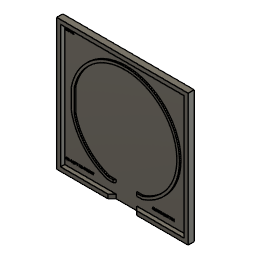
pin_grid_center_wafer_jig (Autodesk Fusion 360 design; units mm, degrees)
part number: 2026-08-08-01-37-12-857
Autodesk Fusion 360 part; units mm, degrees
ref_plane "WorkPlane1" through (0, 0, 2) normal (0, 0, 1) x (1, 0, 0)
ref_plane "WorkPlane2" through (0, 0, 3.7) normal (0, 0, 1) x (1, 0, 0)
ref_plane "WorkPlane3" through (0, 0, 6.2) normal (0, 0, 1) x (1, 0, 0)
ref_plane "WorkPlane4" through (0, 0, -5) normal (0, 0, 1) x (1, 0, 0)
ref_plane "WorkPlane5" through (0, 0, -4) normal (0, 0, 1) x (1, 0, 0)
sketch "128 mm Square Wafer Platform Sketch" plane through (0, 0, 0) normal (0, 0, 1) x (1, 0, 0)
  line L0 (-56.71, -68.95) -> (71.29, -68.95)
  line L1 (71.29, -68.95) -> (71.29, 59.05)
  line L2 (71.29, 59.05) -> (-56.71, 59.05)
  line L3 (-56.71, 59.05) -> (-56.71, -68.95)
extrude "128 mm Square Wafer Platform" add sketch "128 mm Square Wafer Platform Sketch" along normal blind 2
sketch "4 x 4 mm Perimeter Reinforcement Bar Sketch" plane through (0, 0, 2) normal (0, 0, 1) x (1, 0, 0)
  line L0 (-56.71, -68.95) -> (71.29, -68.95)
  line L1 (71.29, -68.95) -> (71.29, 59.05)
  line L2 (71.29, 59.05) -> (-56.71, 59.05)
  line L3 (-56.71, 59.05) -> (-56.71, -68.95)
  line L4 (-52.71, -64.95) -> (67.29, -64.95)
  line L5 (67.29, -64.95) -> (67.29, 55.05)
  line L6 (67.29, 55.05) -> (-52.71, 55.05)
  line L7 (-52.71, 55.05) -> (-52.71, -64.95)
extrude "4 x 4 mm Perimeter Reinforcement Bar" add sketch "4 x 4 mm Perimeter Reinforcement Bar Sketch" along normal blind 4
sketch "20 mm Outer Bar Tweezer Notch with 45 Degree Sides Lower Sketch" plane through (0, 0, 2) normal (0, 0, 1) x (1, 0, 0)
  line L0 (-2.71, -69.05) -> (17.29, -69.05)
  line L1 (17.29, -69.05) -> (17.29, -64.85)
  line L2 (17.29, -64.85) -> (-2.71, -64.85)
  line L3 (-2.71, -64.85) -> (-2.71, -69.05)
sketch "20 mm Outer Bar Tweezer Notch with 45 Degree Sides Upper Sketch" plane through (0, 0, 6.2) normal (0, 0, 1) x (1, 0, 0)
  line L0 (-6.91, -73.25) -> (21.49, -73.25)
  line L1 (21.49, -73.25) -> (21.49, -60.65)
  line L2 (21.49, -60.65) -> (-6.91, -60.65)
  line L3 (-6.91, -60.65) -> (-6.91, -73.25)
loft "20 mm Outer Bar Tweezer Notch with 45 Degree Sides" cut profiles "20 mm Outer Bar Tweezer Notch with 45 Degree Sides Lower Sketch", "20 mm Outer Bar Tweezer Notch with 45 Degree Sides Upper Sketch" section 1 section 2
sketch "1.5 mm Raised Wafer Nest Sketch" plane through (0, 0, 2) normal (0, 0, 1) x (1, 0, 0)
  line L0 (60.29, -4.95) -> (60.2577, -3.1003)
  line L1 (60.2577, -3.1003) -> (60.1609, -1.2529)
  line L2 (60.1609, -1.2529) -> (59.9997, 0.59)
  line L3 (59.9997, 0.59) -> (59.7742, 2.4262)
  line L4 (59.7742, 2.4262) -> (59.4848, 4.2534)
  line L5 (59.4848, 4.2534) -> (59.1318, 6.0693)
  line L6 (59.1318, 6.0693) -> (58.7157, 7.8719)
  line L7 (58.7157, 7.8719) -> (58.2369, 9.6588)
  line L8 (58.2369, 9.6588) -> (57.696, 11.4279)
  line L9 (57.696, 11.4279) -> (57.0937, 13.1771)
  line L10 (57.0937, 13.1771) -> (56.4307, 14.9041)
  line L11 (56.4307, 14.9041) -> (55.7079, 16.607)
  line L12 (55.7079, 16.607) -> (54.9261, 18.2837)
  line L13 (54.9261, 18.2837) -> (54.0862, 19.932)
  line L14 (54.0862, 19.932) -> (53.1893, 21.55)
  line L15 (53.1893, 21.55) -> (52.2365, 23.1357)
  line L16 (52.2365, 23.1357) -> (51.229, 24.6872)
  line L17 (51.229, 24.6872) -> (50.1679, 26.2026)
  line L18 (50.1679, 26.2026) -> (49.0546, 27.6801)
  line L19 (49.0546, 27.6801) -> (47.8904, 29.1177)
  line L20 (47.8904, 29.1177) -> (46.6767, 30.5139)
  line L21 (46.6767, 30.5139) -> (45.415, 31.8669)
  line L22 (45.415, 31.8669) -> (44.1069, 33.175)
  line L23 (44.1069, 33.175) -> (42.7539, 34.4367)
  line L24 (42.7539, 34.4367) -> (41.3577, 35.6504)
  line L25 (41.3577, 35.6504) -> (39.9201, 36.8146)
  line L26 (39.9201, 36.8146) -> (38.4426, 37.9279)
  line L27 (38.4426, 37.9279) -> (36.9272, 38.989)
  line L28 (36.9272, 38.989) -> (35.3757, 39.9965)
  line L29 (35.3757, 39.9965) -> (33.79, 40.9493)
  line L30 (33.79, 40.9493) -> (32.172, 41.8462)
  line L31 (32.172, 41.8462) -> (30.5237, 42.6861)
  line L32 (30.5237, 42.6861) -> (28.847, 43.4679)
  line L33 (28.847, 43.4679) -> (27.1441, 44.1907)
  line L34 (27.1441, 44.1907) -> (25.4171, 44.8537)
  line L35 (25.4171, 44.8537) -> (23.6679, 45.456)
  line L36 (23.6679, 45.456) -> (21.8988, 45.9969)
  line L37 (21.8988, 45.9969) -> (20.1119, 46.4757)
  line L38 (20.1119, 46.4757) -> (18.3093, 46.8918)
  line L39 (18.3093, 46.8918) -> (16.4934, 47.2448)
  line L40 (16.4934, 47.2448) -> (14.6662, 47.5342)
  line L41 (14.6662, 47.5342) -> (12.83, 47.7597)
  line L42 (12.83, 47.7597) -> (10.9871, 47.9209)
  line L43 (10.9871, 47.9209) -> (9.1397, 48.0177)
  line L44 (9.1397, 48.0177) -> (7.29, 48.05)
  line L45 (7.29, 48.05) -> (5.4403, 48.0177)
  line L46 (5.4403, 48.0177) -> (3.5929, 47.9209)
  line L47 (3.5929, 47.9209) -> (1.75, 47.7597)
  line L48 (1.75, 47.7597) -> (-0.0862, 47.5342)
  line L49 (-0.0862, 47.5342) -> (-1.9134, 47.2448)
  line L50 (-1.9134, 47.2448) -> (-3.7293, 46.8918)
  line L51 (-3.7293, 46.8918) -> (-5.5319, 46.4757)
  line L52 (-5.5319, 46.4757) -> (-7.3188, 45.9969)
  line L53 (-7.3188, 45.9969) -> (-9.0879, 45.456)
  line L54 (-9.0879, 45.456) -> (-10.8371, 44.8537)
  line L55 (-10.8371, 44.8537) -> (-12.5641, 44.1907)
  line L56 (-12.5641, 44.1907) -> (-14.267, 43.4679)
  line L57 (-14.267, 43.4679) -> (-15.9437, 42.6861)
  line L58 (-15.9437, 42.6861) -> (-17.592, 41.8462)
  line L59 (-17.592, 41.8462) -> (-19.21, 40.9493)
  line L60 (-19.21, 40.9493) -> (-20.7957, 39.9965)
  line L61 (-20.7957, 39.9965) -> (-22.3472, 38.989)
  line L62 (-22.3472, 38.989) -> (-23.8626, 37.9279)
  line L63 (-23.8626, 37.9279) -> (-25.3401, 36.8146)
  line L64 (-25.3401, 36.8146) -> (-26.7777, 35.6504)
  line L65 (-26.7777, 35.6504) -> (-28.1739, 34.4367)
  line L66 (-28.1739, 34.4367) -> (-29.5269, 33.175)
  line L67 (-29.5269, 33.175) -> (-30.835, 31.8669)
  line L68 (-30.835, 31.8669) -> (-32.0967, 30.5139)
  line L69 (-32.0967, 30.5139) -> (-33.3104, 29.1177)
  line L70 (-33.3104, 29.1177) -> (-34.4746, 27.6801)
  line L71 (-34.4746, 27.6801) -> (-35.5879, 26.2026)
  line L72 (-35.5879, 26.2026) -> (-36.649, 24.6872)
  line L73 (-36.649, 24.6872) -> (-37.6565, 23.1357)
  line L74 (-37.6565, 23.1357) -> (-38.6093, 21.55)
  line L75 (-38.6093, 21.55) -> (-39.5062, 19.932)
  line L76 (-39.5062, 19.932) -> (-40.3461, 18.2837)
  line L77 (-40.3461, 18.2837) -> (-41.1279, 16.607)
  line L78 (-41.1279, 16.607) -> (-41.8507, 14.9041)
  line L79 (-41.8507, 14.9041) -> (-42.5137, 13.1771)
  line L80 (-42.5137, 13.1771) -> (-43.116, 11.4279)
  line L81 (-43.116, 11.4279) -> (-43.6569, 9.6588)
  line L82 (-43.6569, 9.6588) -> (-44.1357, 7.8719)
  line L83 (-44.1357, 7.8719) -> (-44.5518, 6.0693)
  line L84 (-44.5518, 6.0693) -> (-44.8933, 4.3124)
  line L85 (-44.8933, 4.3124) -> (-44.8933, -14.2124)
  line L86 (-44.8933, -14.2124) -> (-44.5518, -15.9693)
  line L87 (-44.5518, -15.9693) -> (-44.1357, -17.7719)
  line L88 (-44.1357, -17.7719) -> (-43.6569, -19.5588)
  line L89 (-43.6569, -19.5588) -> (-43.116, -21.3279)
  line L90 (-43.116, -21.3279) -> (-42.5137, -23.0771)
  line L91 (-42.5137, -23.0771) -> (-41.8507, -24.8041)
  line L92 (-41.8507, -24.8041) -> (-41.1279, -26.507)
  line L93 (-41.1279, -26.507) -> (-40.3461, -28.1837)
  line L94 (-40.3461, -28.1837) -> (-39.5062, -29.832)
  line L95 (-39.5062, -29.832) -> (-38.6093, -31.45)
  line L96 (-38.6093, -31.45) -> (-37.6565, -33.0357)
  line L97 (-37.6565, -33.0357) -> (-36.649, -34.5872)
  line L98 (-36.649, -34.5872) -> (-35.5879, -36.1026)
  line L99 (-35.5879, -36.1026) -> (-34.4746, -37.5801)
  line L100 (-34.4746, -37.5801) -> (-33.3104, -39.0177)
  line L101 (-33.3104, -39.0177) -> (-32.0967, -40.4139)
  line L102 (-32.0967, -40.4139) -> (-30.835, -41.7669)
  line L103 (-30.835, -41.7669) -> (-29.5269, -43.075)
  line L104 (-29.5269, -43.075) -> (-28.1739, -44.3367)
  line L105 (-28.1739, -44.3367) -> (-26.7777, -45.5504)
  line L106 (-26.7777, -45.5504) -> (-25.3401, -46.7146)
  line L107 (-25.3401, -46.7146) -> (-23.8626, -47.8279)
  line L108 (-23.8626, -47.8279) -> (-22.3472, -48.889)
  line L109 (-22.3472, -48.889) -> (-20.7957, -49.8965)
  line L110 (-20.7957, -49.8965) -> (-19.21, -50.8493)
  line L111 (-19.21, -50.8493) -> (-17.592, -51.7462)
  line L112 (-17.592, -51.7462) -> (-15.9437, -52.5861)
  line L113 (-15.9437, -52.5861) -> (-14.267, -53.3679)
  line L114 (-14.267, -53.3679) -> (-12.5641, -54.0907)
  line L115 (-12.5641, -54.0907) -> (-10.8371, -54.7537)
  line L116 (-10.8371, -54.7537) -> (-9.4373, -55.2357)
  line L117 (-9.4373, -55.2357) -> (24.0173, -55.2357)
  line L118 (24.0173, -55.2357) -> (25.4171, -54.7537)
  line L119 (25.4171, -54.7537) -> (27.1441, -54.0907)
  line L120 (27.1441, -54.0907) -> (28.847, -53.3679)
  line L121 (28.847, -53.3679) -> (30.5237, -52.5861)
  line L122 (30.5237, -52.5861) -> (32.172, -51.7462)
  line L123 (32.172, -51.7462) -> (33.79, -50.8493)
  line L124 (33.79, -50.8493) -> (35.3757, -49.8965)
  line L125 (35.3757, -49.8965) -> (36.9272, -48.889)
  line L126 (36.9272, -48.889) -> (38.4426, -47.8279)
  line L127 (38.4426, -47.8279) -> (39.9201, -46.7146)
  line L128 (39.9201, -46.7146) -> (41.3577, -45.5504)
  line L129 (41.3577, -45.5504) -> (42.7539, -44.3367)
  line L130 (42.7539, -44.3367) -> (44.1069, -43.075)
  line L131 (44.1069, -43.075) -> (45.415, -41.7669)
  line L132 (45.415, -41.7669) -> (46.6767, -40.4139)
  line L133 (46.6767, -40.4139) -> (47.8904, -39.0177)
  line L134 (47.8904, -39.0177) -> (49.0546, -37.5801)
  line L135 (49.0546, -37.5801) -> (50.1679, -36.1026)
  line L136 (50.1679, -36.1026) -> (51.229, -34.5872)
  line L137 (51.229, -34.5872) -> (52.2365, -33.0357)
  line L138 (52.2365, -33.0357) -> (53.1893, -31.45)
  line L139 (53.1893, -31.45) -> (54.0862, -29.832)
  line L140 (54.0862, -29.832) -> (54.9261, -28.1837)
  line L141 (54.9261, -28.1837) -> (55.7079, -26.507)
  line L142 (55.7079, -26.507) -> (56.4307, -24.8041)
  line L143 (56.4307, -24.8041) -> (57.0937, -23.0771)
  line L144 (57.0937, -23.0771) -> (57.696, -21.3279)
  line L145 (57.696, -21.3279) -> (58.2369, -19.5588)
  line L146 (58.2369, -19.5588) -> (58.7157, -17.7719)
  line L147 (58.7157, -17.7719) -> (59.1318, -15.9693)
  line L148 (59.1318, -15.9693) -> (59.4848, -14.1534)
  line L149 (59.4848, -14.1534) -> (59.7742, -12.3262)
  line L150 (59.7742, -12.3262) -> (59.9997, -10.49)
  line L151 (59.9997, -10.49) -> (60.1609, -8.6471)
  line L152 (60.1609, -8.6471) -> (60.2577, -6.7997)
  line L153 (60.2577, -6.7997) -> (60.29, -4.95)
extrude "1.5 mm Raised Wafer Nest" add sketch "1.5 mm Raised Wafer Nest Sketch" along normal blind 1.5
sketch "Final Wafer Pocket Clearance Sketch" plane through (0, 0, 2) normal (0, 0, 1) x (1, 0, 0)
  line L0 (57.79, -4.95) -> (57.7592, -3.1876)
  line L1 (57.7592, -3.1876) -> (57.667, -1.4273)
  line L2 (57.667, -1.4273) -> (57.5134, 0.3287)
  line L3 (57.5134, 0.3287) -> (57.2985, 2.0782)
  line L4 (57.2985, 2.0782) -> (57.0228, 3.8192)
  line L5 (57.0228, 3.8192) -> (56.6865, 5.5495)
  line L6 (56.6865, 5.5495) -> (56.2899, 7.2671)
  line L7 (56.2899, 7.2671) -> (55.8337, 8.9697)
  line L8 (55.8337, 8.9697) -> (55.3184, 10.6554)
  line L9 (55.3184, 10.6554) -> (54.7445, 12.322)
  line L10 (54.7445, 12.322) -> (54.1128, 13.9676)
  line L11 (54.1128, 13.9676) -> (53.424, 15.5902)
  line L12 (53.424, 15.5902) -> (52.6791, 17.1877)
  line L13 (52.6791, 17.1877) -> (51.8789, 18.7583)
  line L14 (51.8789, 18.7583) -> (51.0243, 20.3)
  line L15 (51.0243, 20.3) -> (50.1164, 21.8109)
  line L16 (50.1164, 21.8109) -> (49.1564, 23.2892)
  line L17 (49.1564, 23.2892) -> (48.1454, 24.7332)
  line L18 (48.1454, 24.7332) -> (47.0845, 26.1409)
  line L19 (47.0845, 26.1409) -> (45.9752, 27.5108)
  line L20 (45.9752, 27.5108) -> (44.8188, 28.8411)
  line L21 (44.8188, 28.8411) -> (43.6167, 30.1302)
  line L22 (43.6167, 30.1302) -> (42.3702, 31.3767)
  line L23 (42.3702, 31.3767) -> (41.0811, 32.5788)
  line L24 (41.0811, 32.5788) -> (39.7508, 33.7352)
  line L25 (39.7508, 33.7352) -> (38.3809, 34.8445)
  line L26 (38.3809, 34.8445) -> (36.9732, 35.9054)
  line L27 (36.9732, 35.9054) -> (35.5292, 36.9164)
  line L28 (35.5292, 36.9164) -> (34.0509, 37.8764)
  line L29 (34.0509, 37.8764) -> (32.54, 38.7843)
  line L30 (32.54, 38.7843) -> (30.9983, 39.6389)
  line L31 (30.9983, 39.6389) -> (29.4277, 40.4391)
  line L32 (29.4277, 40.4391) -> (27.8302, 41.184)
  line L33 (27.8302, 41.184) -> (26.2076, 41.8728)
  line L34 (26.2076, 41.8728) -> (24.562, 42.5045)
  line L35 (24.562, 42.5045) -> (22.8954, 43.0784)
  line L36 (22.8954, 43.0784) -> (21.2097, 43.5937)
  line L37 (21.2097, 43.5937) -> (19.5071, 44.0499)
  line L38 (19.5071, 44.0499) -> (17.7895, 44.4465)
  line L39 (17.7895, 44.4465) -> (16.0592, 44.7828)
  line L40 (16.0592, 44.7828) -> (14.3182, 45.0585)
  line L41 (14.3182, 45.0585) -> (12.5687, 45.2734)
  line L42 (12.5687, 45.2734) -> (10.8127, 45.427)
  line L43 (10.8127, 45.427) -> (9.0524, 45.5192)
  line L44 (9.0524, 45.5192) -> (7.29, 45.55)
  line L45 (7.29, 45.55) -> (5.5276, 45.5192)
  line L46 (5.5276, 45.5192) -> (3.7673, 45.427)
  line L47 (3.7673, 45.427) -> (2.0113, 45.2734)
  line L48 (2.0113, 45.2734) -> (0.2618, 45.0585)
  line L49 (0.2618, 45.0585) -> (-1.4792, 44.7828)
  line L50 (-1.4792, 44.7828) -> (-3.2095, 44.4465)
  line L51 (-3.2095, 44.4465) -> (-4.9271, 44.0499)
  line L52 (-4.9271, 44.0499) -> (-6.6297, 43.5937)
  line L53 (-6.6297, 43.5937) -> (-8.3154, 43.0784)
  line L54 (-8.3154, 43.0784) -> (-9.982, 42.5045)
  line L55 (-9.982, 42.5045) -> (-11.6276, 41.8728)
  line L56 (-11.6276, 41.8728) -> (-13.2502, 41.184)
  line L57 (-13.2502, 41.184) -> (-14.8477, 40.4391)
  line L58 (-14.8477, 40.4391) -> (-16.4183, 39.6389)
  line L59 (-16.4183, 39.6389) -> (-17.96, 38.7843)
  line L60 (-17.96, 38.7843) -> (-19.4709, 37.8764)
  line L61 (-19.4709, 37.8764) -> (-20.9492, 36.9164)
  line L62 (-20.9492, 36.9164) -> (-22.3932, 35.9054)
  line L63 (-22.3932, 35.9054) -> (-23.8009, 34.8445)
  line L64 (-23.8009, 34.8445) -> (-25.1708, 33.7352)
  line L65 (-25.1708, 33.7352) -> (-26.5011, 32.5788)
  line L66 (-26.5011, 32.5788) -> (-27.7902, 31.3767)
  line L67 (-27.7902, 31.3767) -> (-29.0367, 30.1302)
  line L68 (-29.0367, 30.1302) -> (-30.2388, 28.8411)
  line L69 (-30.2388, 28.8411) -> (-31.3952, 27.5108)
  line L70 (-31.3952, 27.5108) -> (-32.5045, 26.1409)
  line L71 (-32.5045, 26.1409) -> (-33.5654, 24.7332)
  line L72 (-33.5654, 24.7332) -> (-34.5764, 23.2892)
  line L73 (-34.5764, 23.2892) -> (-35.5364, 21.8109)
  line L74 (-35.5364, 21.8109) -> (-36.4443, 20.3)
  line L75 (-36.4443, 20.3) -> (-37.2989, 18.7583)
  line L76 (-37.2989, 18.7583) -> (-38.0991, 17.1877)
  line L77 (-38.0991, 17.1877) -> (-38.844, 15.5902)
  line L78 (-38.844, 15.5902) -> (-39.5328, 13.9676)
  line L79 (-39.5328, 13.9676) -> (-40.1645, 12.322)
  line L80 (-40.1645, 12.322) -> (-40.7384, 10.6554)
  line L81 (-40.7384, 10.6554) -> (-41.2537, 8.9697)
  line L82 (-41.2537, 8.9697) -> (-41.7099, 7.2671)
  line L83 (-41.7099, 7.2671) -> (-41.9933, 6.0395)
  line L84 (-41.9933, 6.0395) -> (-41.9933, -15.9395)
  line L85 (-41.9933, -15.9395) -> (-41.7099, -17.1671)
  line L86 (-41.7099, -17.1671) -> (-41.2537, -18.8697)
  line L87 (-41.2537, -18.8697) -> (-40.7384, -20.5554)
  line L88 (-40.7384, -20.5554) -> (-40.1645, -22.222)
  line L89 (-40.1645, -22.222) -> (-39.5328, -23.8676)
  line L90 (-39.5328, -23.8676) -> (-38.844, -25.4902)
  line L91 (-38.844, -25.4902) -> (-38.0991, -27.0877)
  line L92 (-38.0991, -27.0877) -> (-37.2989, -28.6583)
  line L93 (-37.2989, -28.6583) -> (-36.4443, -30.2)
  line L94 (-36.4443, -30.2) -> (-35.5364, -31.7109)
  line L95 (-35.5364, -31.7109) -> (-34.5764, -33.1892)
  line L96 (-34.5764, -33.1892) -> (-33.5654, -34.6332)
  line L97 (-33.5654, -34.6332) -> (-32.5045, -36.0409)
  line L98 (-32.5045, -36.0409) -> (-31.3952, -37.4108)
  line L99 (-31.3952, -37.4108) -> (-30.2388, -38.7411)
  line L100 (-30.2388, -38.7411) -> (-29.0367, -40.0302)
  line L101 (-29.0367, -40.0302) -> (-27.7902, -41.2767)
  line L102 (-27.7902, -41.2767) -> (-26.5011, -42.4788)
  line L103 (-26.5011, -42.4788) -> (-25.1708, -43.6352)
  line L104 (-25.1708, -43.6352) -> (-23.8009, -44.7445)
  line L105 (-23.8009, -44.7445) -> (-22.3932, -45.8054)
  line L106 (-22.3932, -45.8054) -> (-20.9492, -46.8164)
  line L107 (-20.9492, -46.8164) -> (-19.4709, -47.7764)
  line L108 (-19.4709, -47.7764) -> (-17.96, -48.6843)
  line L109 (-17.96, -48.6843) -> (-16.4183, -49.5389)
  line L110 (-16.4183, -49.5389) -> (-14.8477, -50.3391)
  line L111 (-14.8477, -50.3391) -> (-13.2502, -51.084)
  line L112 (-13.2502, -51.084) -> (-11.6276, -51.7728)
  line L113 (-11.6276, -51.7728) -> (-9.982, -52.4045)
  line L114 (-9.982, -52.4045) -> (-9.0201, -52.7357)
  line L115 (-9.0201, -52.7357) -> (23.6001, -52.7357)
  line L116 (23.6001, -52.7357) -> (24.562, -52.4045)
  line L117 (24.562, -52.4045) -> (26.2076, -51.7728)
  line L118 (26.2076, -51.7728) -> (27.8302, -51.084)
  line L119 (27.8302, -51.084) -> (29.4277, -50.3391)
  line L120 (29.4277, -50.3391) -> (30.9983, -49.5389)
  line L121 (30.9983, -49.5389) -> (32.54, -48.6843)
  line L122 (32.54, -48.6843) -> (34.0509, -47.7764)
  line L123 (34.0509, -47.7764) -> (35.5292, -46.8164)
  line L124 (35.5292, -46.8164) -> (36.9732, -45.8054)
  line L125 (36.9732, -45.8054) -> (38.3809, -44.7445)
  line L126 (38.3809, -44.7445) -> (39.7508, -43.6352)
  line L127 (39.7508, -43.6352) -> (41.0811, -42.4788)
  line L128 (41.0811, -42.4788) -> (42.3702, -41.2767)
  line L129 (42.3702, -41.2767) -> (43.6167, -40.0302)
  line L130 (43.6167, -40.0302) -> (44.8188, -38.7411)
  line L131 (44.8188, -38.7411) -> (45.9752, -37.4108)
  line L132 (45.9752, -37.4108) -> (47.0845, -36.0409)
  line L133 (47.0845, -36.0409) -> (48.1454, -34.6332)
  line L134 (48.1454, -34.6332) -> (49.1564, -33.1892)
  line L135 (49.1564, -33.1892) -> (50.1164, -31.7109)
  line L136 (50.1164, -31.7109) -> (51.0243, -30.2)
  line L137 (51.0243, -30.2) -> (51.8789, -28.6583)
  line L138 (51.8789, -28.6583) -> (52.6791, -27.0877)
  line L139 (52.6791, -27.0877) -> (53.424, -25.4902)
  line L140 (53.424, -25.4902) -> (54.1128, -23.8676)
  line L141 (54.1128, -23.8676) -> (54.7445, -22.222)
  line L142 (54.7445, -22.222) -> (55.3184, -20.5554)
  line L143 (55.3184, -20.5554) -> (55.8337, -18.8697)
  line L144 (55.8337, -18.8697) -> (56.2899, -17.1671)
  line L145 (56.2899, -17.1671) -> (56.6865, -15.4495)
  line L146 (56.6865, -15.4495) -> (57.0228, -13.7192)
  line L147 (57.0228, -13.7192) -> (57.2985, -11.9782)
  line L148 (57.2985, -11.9782) -> (57.5134, -10.2287)
  line L149 (57.5134, -10.2287) -> (57.667, -8.4727)
  line L150 (57.667, -8.4727) -> (57.7592, -6.7124)
  line L151 (57.7592, -6.7124) -> (57.79, -4.95)
extrude "Final Wafer Pocket Clearance" cut sketch "Final Wafer Pocket Clearance Sketch" along normal blind 1.6
sketch "20 mm Pickup Opening with 45 Degree Bevel Lower Sketch" plane through (0, 0, 2) normal (0, 0, 1) x (1, 0, 0)
  line L0 (-2.71, -55.2357) -> (-2.71, -52.2357)
  line L1 (-2.71, -52.2357) -> (-2.6471, -51.1161)
  line L2 (-2.6471, -51.1161) -> (-2.4593, -50.0105)
  line L3 (-2.4593, -50.0105) -> (-2.1488, -48.9329)
  line L4 (-2.1488, -48.9329) -> (-1.7197, -47.8969)
  line L5 (-1.7197, -47.8969) -> (-1.1772, -46.9154)
  line L6 (-1.1772, -46.9154) -> (-0.5283, -46.0008)
  line L7 (-0.5283, -46.0008) -> (0.2189, -45.1646)
  line L8 (0.2189, -45.1646) -> (1.0551, -44.4174)
  line L9 (1.0551, -44.4174) -> (1.9697, -43.7685)
  line L10 (1.9697, -43.7685) -> (2.9512, -43.226)
  line L11 (2.9512, -43.226) -> (3.9872, -42.7969)
  line L12 (3.9872, -42.7969) -> (5.0648, -42.4864)
  line L13 (5.0648, -42.4864) -> (6.1704, -42.2986)
  line L14 (6.1704, -42.2986) -> (7.29, -42.2357)
  line L15 (7.29, -42.2357) -> (8.4096, -42.2986)
  line L16 (8.4096, -42.2986) -> (9.5152, -42.4864)
  line L17 (9.5152, -42.4864) -> (10.5928, -42.7969)
  line L18 (10.5928, -42.7969) -> (11.6288, -43.226)
  line L19 (11.6288, -43.226) -> (12.6103, -43.7685)
  line L20 (12.6103, -43.7685) -> (13.5249, -44.4174)
  line L21 (13.5249, -44.4174) -> (14.3611, -45.1646)
  line L22 (14.3611, -45.1646) -> (15.1083, -46.0008)
  line L23 (15.1083, -46.0008) -> (15.7572, -46.9154)
  line L24 (15.7572, -46.9154) -> (16.2997, -47.8969)
  line L25 (16.2997, -47.8969) -> (16.7288, -48.9329)
  line L26 (16.7288, -48.9329) -> (17.0393, -50.0105)
  line L27 (17.0393, -50.0105) -> (17.2271, -51.1161)
  line L28 (17.2271, -51.1161) -> (17.29, -52.2357)
  line L29 (17.29, -52.2357) -> (17.29, -55.2357)
  line L30 (17.29, -55.2357) -> (17.2271, -56.3553)
  line L31 (17.2271, -56.3553) -> (17.0393, -57.4609)
  line L32 (17.0393, -57.4609) -> (16.7288, -58.5385)
  line L33 (16.7288, -58.5385) -> (16.2997, -59.5745)
  line L34 (16.2997, -59.5745) -> (15.7572, -60.556)
  line L35 (15.7572, -60.556) -> (15.1083, -61.4706)
  line L36 (15.1083, -61.4706) -> (14.3611, -62.3068)
  line L37 (14.3611, -62.3068) -> (13.5249, -63.054)
  line L38 (13.5249, -63.054) -> (12.6103, -63.7029)
  line L39 (12.6103, -63.7029) -> (11.6288, -64.2454)
  line L40 (11.6288, -64.2454) -> (10.5928, -64.6745)
  line L41 (10.5928, -64.6745) -> (9.5152, -64.985)
  line L42 (9.5152, -64.985) -> (8.4096, -65.1728)
  line L43 (8.4096, -65.1728) -> (7.29, -65.2357)
  line L44 (7.29, -65.2357) -> (6.1704, -65.1728)
  line L45 (6.1704, -65.1728) -> (5.0648, -64.985)
  line L46 (5.0648, -64.985) -> (3.9872, -64.6745)
  line L47 (3.9872, -64.6745) -> (2.9512, -64.2454)
  line L48 (2.9512, -64.2454) -> (1.9697, -63.7029)
  line L49 (1.9697, -63.7029) -> (1.0551, -63.054)
  line L50 (1.0551, -63.054) -> (0.2189, -62.3068)
  line L51 (0.2189, -62.3068) -> (-0.5283, -61.4706)
  line L52 (-0.5283, -61.4706) -> (-1.1772, -60.556)
  line L53 (-1.1772, -60.556) -> (-1.7197, -59.5745)
  line L54 (-1.7197, -59.5745) -> (-2.1488, -58.5385)
  line L55 (-2.1488, -58.5385) -> (-2.4593, -57.4609)
  line L56 (-2.4593, -57.4609) -> (-2.6471, -56.3553)
  line L57 (-2.6471, -56.3553) -> (-2.71, -55.2357)
sketch "20 mm Pickup Opening with 45 Degree Bevel Upper Sketch" plane through (0, 0, 3.7) normal (0, 0, 1) x (1, 0, 0)
  line L0 (-4.41, -56.9357) -> (-4.41, -50.5357)
  line L1 (-4.41, -50.5357) -> (-4.3364, -49.2257)
  line L2 (-4.3364, -49.2257) -> (-4.1167, -47.9322)
  line L3 (-4.1167, -47.9322) -> (-3.7534, -46.6714)
  line L4 (-3.7534, -46.6714) -> (-3.2513, -45.4593)
  line L5 (-3.2513, -45.4593) -> (-2.6167, -44.3109)
  line L6 (-2.6167, -44.3109) -> (-1.8574, -43.2409)
  line L7 (-1.8574, -43.2409) -> (-0.9831, -42.2626)
  line L8 (-0.9831, -42.2626) -> (-0.0048, -41.3883)
  line L9 (-0.0048, -41.3883) -> (1.0652, -40.629)
  line L10 (1.0652, -40.629) -> (2.2136, -39.9944)
  line L11 (2.2136, -39.9944) -> (3.4257, -39.4923)
  line L12 (3.4257, -39.4923) -> (4.6865, -39.129)
  line L13 (4.6865, -39.129) -> (5.98, -38.9093)
  line L14 (5.98, -38.9093) -> (7.29, -38.8357)
  line L15 (7.29, -38.8357) -> (8.6, -38.9093)
  line L16 (8.6, -38.9093) -> (9.8935, -39.129)
  line L17 (9.8935, -39.129) -> (11.1543, -39.4923)
  line L18 (11.1543, -39.4923) -> (12.3664, -39.9944)
  line L19 (12.3664, -39.9944) -> (13.5148, -40.629)
  line L20 (13.5148, -40.629) -> (14.5848, -41.3883)
  line L21 (14.5848, -41.3883) -> (15.5631, -42.2626)
  line L22 (15.5631, -42.2626) -> (16.4374, -43.2409)
  line L23 (16.4374, -43.2409) -> (17.1967, -44.3109)
  line L24 (17.1967, -44.3109) -> (17.8313, -45.4593)
  line L25 (17.8313, -45.4593) -> (18.3334, -46.6714)
  line L26 (18.3334, -46.6714) -> (18.6967, -47.9322)
  line L27 (18.6967, -47.9322) -> (18.9164, -49.2257)
  line L28 (18.9164, -49.2257) -> (18.99, -50.5357)
  line L29 (18.99, -50.5357) -> (18.99, -56.9357)
  line L30 (18.99, -56.9357) -> (18.9164, -58.2457)
  line L31 (18.9164, -58.2457) -> (18.6967, -59.5392)
  line L32 (18.6967, -59.5392) -> (18.3334, -60.8)
  line L33 (18.3334, -60.8) -> (17.8313, -62.0121)
  line L34 (17.8313, -62.0121) -> (17.1967, -63.1605)
  line L35 (17.1967, -63.1605) -> (16.4374, -64.2305)
  line L36 (16.4374, -64.2305) -> (15.5631, -65.2089)
  line L37 (15.5631, -65.2089) -> (14.5848, -66.0831)
  line L38 (14.5848, -66.0831) -> (13.5148, -66.8424)
  line L39 (13.5148, -66.8424) -> (12.3664, -67.477)
  line L40 (12.3664, -67.477) -> (11.1543, -67.9791)
  line L41 (11.1543, -67.9791) -> (9.8935, -68.3424)
  line L42 (9.8935, -68.3424) -> (8.6, -68.5621)
  line L43 (8.6, -68.5621) -> (7.29, -68.6357)
  line L44 (7.29, -68.6357) -> (5.98, -68.5621)
  line L45 (5.98, -68.5621) -> (4.6865, -68.3424)
  line L46 (4.6865, -68.3424) -> (3.4257, -67.9791)
  line L47 (3.4257, -67.9791) -> (2.2136, -67.477)
  line L48 (2.2136, -67.477) -> (1.0652, -66.8424)
  line L49 (1.0652, -66.8424) -> (-0.0048, -66.0831)
  line L50 (-0.0048, -66.0831) -> (-0.9831, -65.2089)
  line L51 (-0.9831, -65.2089) -> (-1.8574, -64.2305)
  line L52 (-1.8574, -64.2305) -> (-2.6167, -63.1605)
  line L53 (-2.6167, -63.1605) -> (-3.2513, -62.0121)
  line L54 (-3.2513, -62.0121) -> (-3.7534, -60.8)
  line L55 (-3.7534, -60.8) -> (-4.1167, -59.5392)
  line L56 (-4.1167, -59.5392) -> (-4.3364, -58.2457)
  line L57 (-4.3364, -58.2457) -> (-4.41, -56.9357)
loft "20 mm Pickup Opening with 45 Degree Bevel" cut profiles "20 mm Pickup Opening with 45 Degree Bevel Lower Sketch", "20 mm Pickup Opening with 45 Degree Bevel Upper Sketch" section 1 section 2
sketch "Outer Front Left Pin Cylinder Sketch" plane through (0, 0, -4) normal (0, 0, 1) x (1, 0, 0)
  circle A0 centre (-50.8, -50.8) radius 2.35
extrude "Outer Front Left 4.7 mm Pin" add sketch "Outer Front Left Pin Cylinder Sketch" along normal blind 6
sketch "Outer Front Left Tapered Tip Tip" plane through (0, 0, -5) normal (0, 0, 1) x (1, 0, 0)
  circle A0 centre (-50.8, -50.8) radius 2
sketch "Outer Front Left Tapered Tip Shoulder" plane through (0, 0, -4) normal (0, 0, 1) x (1, 0, 0)
  circle A0 centre (-50.8, -50.8) radius 2.35
loft "Outer Front Left Tapered Tip" add profiles "Outer Front Left Tapered Tip Tip", "Outer Front Left Tapered Tip Shoulder" section 1 section 2
sketch "Outer Front Right Pin Cylinder Sketch" plane through (0, 0, -4) normal (0, 0, 1) x (1, 0, 0)
  circle A0 centre (50.8, -50.8) radius 2.35
extrude "Outer Front Right 4.7 mm Pin" add sketch "Outer Front Right Pin Cylinder Sketch" along normal blind 6
sketch "Outer Front Right Tapered Tip Tip" plane through (0, 0, -5) normal (0, 0, 1) x (1, 0, 0)
  circle A0 centre (50.8, -50.8) radius 2
sketch "Outer Front Right Tapered Tip Shoulder" plane through (0, 0, -4) normal (0, 0, 1) x (1, 0, 0)
  circle A0 centre (50.8, -50.8) radius 2.35
loft "Outer Front Right Tapered Tip" add profiles "Outer Front Right Tapered Tip Tip", "Outer Front Right Tapered Tip Shoulder" section 1 section 2
sketch "Outer Rear Left Pin Cylinder Sketch" plane through (0, 0, -4) normal (0, 0, 1) x (1, 0, 0)
  circle A0 centre (-50.8, 50.8) radius 2.35
extrude "Outer Rear Left 4.7 mm Pin" add sketch "Outer Rear Left Pin Cylinder Sketch" along normal blind 6
sketch "Outer Rear Left Tapered Tip Tip" plane through (0, 0, -5) normal (0, 0, 1) x (1, 0, 0)
  circle A0 centre (-50.8, 50.8) radius 2
sketch "Outer Rear Left Tapered Tip Shoulder" plane through (0, 0, -4) normal (0, 0, 1) x (1, 0, 0)
  circle A0 centre (-50.8, 50.8) radius 2.35
loft "Outer Rear Left Tapered Tip" add profiles "Outer Rear Left Tapered Tip Tip", "Outer Rear Left Tapered Tip Shoulder" section 1 section 2
sketch "Outer Rear Right Pin Cylinder Sketch" plane through (0, 0, -4) normal (0, 0, 1) x (1, 0, 0)
  circle A0 centre (50.8, 50.8) radius 2.35
extrude "Outer Rear Right 4.7 mm Pin" add sketch "Outer Rear Right Pin Cylinder Sketch" along normal blind 6
sketch "Outer Rear Right Tapered Tip Tip" plane through (0, 0, -5) normal (0, 0, 1) x (1, 0, 0)
  circle A0 centre (50.8, 50.8) radius 2
sketch "Outer Rear Right Tapered Tip Shoulder" plane through (0, 0, -4) normal (0, 0, 1) x (1, 0, 0)
  circle A0 centre (50.8, 50.8) radius 2.35
loft "Outer Rear Right Tapered Tip" add profiles "Outer Rear Right Tapered Tip Tip", "Outer Rear Right Tapered Tip Shoulder" section 1 section 2
sketch "Inner Front Left Pin Cylinder Sketch" plane through (0, 0, -4) normal (0, 0, 1) x (1, 0, 0)
  circle A0 centre (-25.4, -25.4) radius 2.35
extrude "Inner Front Left 4.7 mm Pin" add sketch "Inner Front Left Pin Cylinder Sketch" along normal blind 6
sketch "Inner Front Left Tapered Tip Tip" plane through (0, 0, -5) normal (0, 0, 1) x (1, 0, 0)
  circle A0 centre (-25.4, -25.4) radius 2
sketch "Inner Front Left Tapered Tip Shoulder" plane through (0, 0, -4) normal (0, 0, 1) x (1, 0, 0)
  circle A0 centre (-25.4, -25.4) radius 2.35
loft "Inner Front Left Tapered Tip" add profiles "Inner Front Left Tapered Tip Tip", "Inner Front Left Tapered Tip Shoulder" section 1 section 2
sketch "Inner Front Right Pin Cylinder Sketch" plane through (0, 0, -4) normal (0, 0, 1) x (1, 0, 0)
  circle A0 centre (25.4, -25.4) radius 2.35
extrude "Inner Front Right 4.7 mm Pin" add sketch "Inner Front Right Pin Cylinder Sketch" along normal blind 6
sketch "Inner Front Right Tapered Tip Tip" plane through (0, 0, -5) normal (0, 0, 1) x (1, 0, 0)
  circle A0 centre (25.4, -25.4) radius 2
sketch "Inner Front Right Tapered Tip Shoulder" plane through (0, 0, -4) normal (0, 0, 1) x (1, 0, 0)
  circle A0 centre (25.4, -25.4) radius 2.35
loft "Inner Front Right Tapered Tip" add profiles "Inner Front Right Tapered Tip Tip", "Inner Front Right Tapered Tip Shoulder" section 1 section 2
sketch "Inner Rear Left Pin Cylinder Sketch" plane through (0, 0, -4) normal (0, 0, 1) x (1, 0, 0)
  circle A0 centre (-25.4, 25.4) radius 2.35
extrude "Inner Rear Left 4.7 mm Pin" add sketch "Inner Rear Left Pin Cylinder Sketch" along normal blind 6
sketch "Inner Rear Left Tapered Tip Tip" plane through (0, 0, -5) normal (0, 0, 1) x (1, 0, 0)
  circle A0 centre (-25.4, 25.4) radius 2
sketch "Inner Rear Left Tapered Tip Shoulder" plane through (0, 0, -4) normal (0, 0, 1) x (1, 0, 0)
  circle A0 centre (-25.4, 25.4) radius 2.35
loft "Inner Rear Left Tapered Tip" add profiles "Inner Rear Left Tapered Tip Tip", "Inner Rear Left Tapered Tip Shoulder" section 1 section 2
sketch "Inner Rear Right Pin Cylinder Sketch" plane through (0, 0, -4) normal (0, 0, 1) x (1, 0, 0)
  circle A0 centre (25.4, 25.4) radius 2.35
extrude "Inner Rear Right 4.7 mm Pin" add sketch "Inner Rear Right Pin Cylinder Sketch" along normal blind 6
sketch "Inner Rear Right Tapered Tip Tip" plane through (0, 0, -5) normal (0, 0, 1) x (1, 0, 0)
  circle A0 centre (25.4, 25.4) radius 2
sketch "Inner Rear Right Tapered Tip Shoulder" plane through (0, 0, -4) normal (0, 0, 1) x (1, 0, 0)
  circle A0 centre (25.4, 25.4) radius 2.35
loft "Inner Rear Right Tapered Tip" add profiles "Inner Rear Right Tapered Tip Tip", "Inner Rear Right Tapered Tip Shoulder" section 1 section 2
sketch "CENTER Position Map - 0.5 mm Engraving Sketch" plane through (0, 0, 2) normal (0, 0, 1) x (1, 0, 0)
  line L0 (-51.71, 44.05) -> (10.29, 44.05) construction
  line L1 (10.29, 44.05) -> (10.29, 54.05) construction
  line L2 (10.29, 54.05) -> (-51.71, 54.05) construction
  line L3 (-51.71, 54.05) -> (-51.71, 44.05) construction
  dimension "d56" = 2
  dimension "d57" = 0
  text T0 "CENTER FIELD ALIGNER\nC5 R2" font "Arial" height 2 align left top in box 62 x 10 at (-51.71, 44.05) x (1, 0) y (0, 1) spacing 1 kerned
extrude "CENTER Position Map - 0.5 mm Engraving" cut sketch "CENTER Position Map - 0.5 mm Engraving Sketch" against normal blind 0.5 text T0
sketch "Grid Orientation Label - 0.5 mm Engraving Sketch" plane through (0, 0, 2) normal (0, 0, 1) x (1, 0, 0)
  line L0 (-51.71, -63.95) -> (-17.71, -63.95) construction
  line L1 (-17.71, -63.95) -> (-17.71, -57.95) construction
  line L2 (-17.71, -57.95) -> (-51.71, -57.95) construction
  line L3 (-51.71, -57.95) -> (-51.71, -63.95) construction
  dimension "d60" = 2
  dimension "d61" = 0
  text T0 "C0=LEFT R0=FRONT" font "Arial" height 2 align left top in box 34 x 6 at (-51.71, -63.95) x (1, 0) y (0, 1) spacing 1 kerned
extrude "Grid Orientation Label - 0.5 mm Engraving" cut sketch "Grid Orientation Label - 0.5 mm Engraving Sketch" against normal blind 0.5 text T0
sketch "Alignment Pin Label - 0.5 mm Engraving Sketch" plane through (0, 0, 2) normal (0, 0, 1) x (1, 0, 0)
  line L0 (32.29, -63.95) -> (66.29, -63.95) construction
  line L1 (66.29, -63.95) -> (66.29, -57.95) construction
  line L2 (66.29, -57.95) -> (32.29, -57.95) construction
  line L3 (32.29, -57.95) -> (32.29, -63.95) construction
  dimension "d64" = 2
  text T0 "ALIGNMENT PIN" font "Arial" height 2 align left top in box 34 x 6 at (32.29, -63.95) x (1, 0) y (0, 1) spacing 1 kerned
extrude "Alignment Pin Label - 0.5 mm Engraving" cut sketch "Alignment Pin Label - 0.5 mm Engraving Sketch" against normal blind 0.5 text T0
equation "gridPitch = 25.4 mm" comment "Table hole-grid pitch"
equation "indexMove = 50.8 mm" comment "Two-grid-space indexing move"
equation "innerPinPatternSpan = 50.8 mm" comment "Two-space inner pin span"
equation "outerPinPatternSpan = 101.6 mm" comment "Four-space outer pin span"
equation "pinDiameter = 4.7 mm" comment "Printed locating pin diameter"
equation "pinEngagement = 5.0 mm" comment "Pin length below platform"
equation "platformSizeX = 128.0 mm" comment "Compact platform width"
equation "platformSizeY = 128.0 mm" comment "Compact platform depth"
equation "baseThickness = 2.0 mm" comment "Wafer platform thickness"
equation "outerBarWidth = 4.0 mm" comment "Perimeter reinforcement width"
equation "outerBarHeight = 4.0 mm" comment "Perimeter reinforcement height"
equation "sidewallHeight = 1.5 mm" comment "Nest lip height above platform"
equation "nestOffsetX = 7.29 mm" comment "Nest X from pin-square center"
equation "nestOffsetY = -4.95 mm" comment "Nest Y from pin-square center"
equation "centerPatternX = 88.89999999999998 mm" comment "Center placement pin-pattern X"
equation "centerPatternY = 114.3 mm" comment "Center placement pin-pattern Y"
equation "centerWaferX = 96.19 mm" comment "Centered wafer X on table"
equation "centerWaferY = 109.35 mm" comment "Centered wafer Y on table"
equation "pickupGapWidth = 20.0 mm" comment "Primary-flat pickup opening"
equation "annotationDepth = 0.5 mm" comment "Baseplate text engraving depth"
equation "annotationTextHeight = 2.0 mm" comment "Baseplate text height"
equation "d57 = 'CENTER FIELD ALIGNER\\nC5 R2'"
equation "d61 = 'C0=LEFT R0=FRONT'"
equation "d65 = 'ALIGNMENT PIN'"
